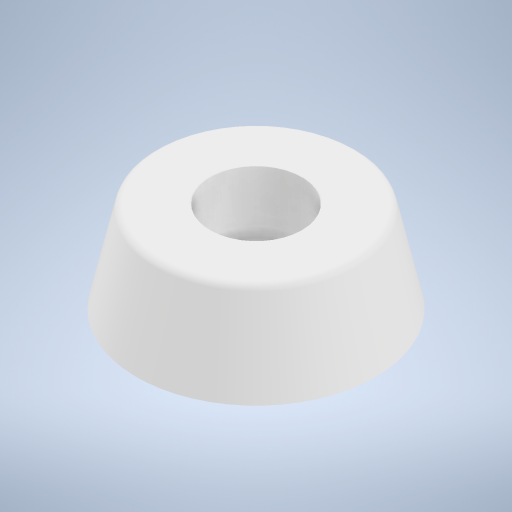
# Autodesk Inventor part: Soft Feet
Saved by Autodesk Inventor 2024 (Build 280153000, 153)
## iProperties
Created: 2023-12-06
Part Number: Soft Feet
Material: Polystyrene, High Impact
Document SubType Name: Modeling
Designer: 18179
Density: 1.022 g/cm^3
Appearance: Smooth - White
Author: 18179
Autodesk Inventor part; units mm, degrees
ref_plane "YZ Plane" through (0, 0, 0) normal (1, 0, 0) x (0, 1, 0)
ref_plane "XY Plane" through (0, 0, 0) normal (0, 0, 1) x (1, 0, 0)
sketch "Sketch1" plane through (0, 0, 0) normal (0, 1, 0) x (-1, 0, 0)
  circle A0 centre (0, 0) radius 12.7
  circle A1 centre (0, 0) radius 2.2225
  dimension "d0" = 25.4
  dimension "d1" = 4.445
  constraints: 2 centre point, 2 coincident
  measures "d0" diameter of A0
  measures "d1" diameter of A1
ref_plane "Work Plane1" through (0, 9.652, 0) normal (0, 1, 0) x (-1, 0, 0)
sketch "Sketch2" plane through (0, 9.652, 0) normal (0, 1, 0) x (-1, 0, 0)
  circle A0 centre (0, 0) radius 2.2238
  circle A1 centre (0, 0) radius 10.541
  dimension "d3" = 21.082
  constraints: 2 centre point, 2 coincident
  measures "d3" diameter of A1
loft "Loft1" add profiles "Sketch1", "Sketch2" contours A0 | A1 / A0 | A1
sketch "Sketch3" plane through (0, 9.652, 0) normal (0, 1, 0) x (1, 0, 0)
  circle A0 centre (0, 0) radius 2.2225
  dimension "d8" = 4.445
  constraints: 1 centre point, 1 coincident
  measures "d8" diameter of A0
extrude "Extrusion1" cut sketch "Sketch3" against normal blind 25.4
sketch "Sketch4" plane through (0, 9.652, 0) normal (0, 1, 0) x (1, 0, 0)
  circle A0 centre (0, 0) radius 4.8895
  dimension "d11" = 9.779
  constraints: 1 centre point, 1 coincident
  measures "d11" diameter of A0
extrude "Extrusion2" cut sketch "Sketch4" against normal blind 6.096
fillet "Fillet1" radius 0.762 2 edges at (10.541, 9.652, 0) (-4.8895, 3.556, 0)
body "Solid1"
